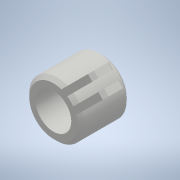
# Autodesk Inventor part: Втулка
Saved by Autodesk Inventor 2020 (Build 240168000, 168)
## iProperties
Created: 2021-05-02
Part Number: Втулка
Material: Типовые
Document SubType Name: Modeling
Designer: I_Love_U_Bogdan
Density: 1 g/cm^3
Appearance: По умолчанию
Author: I_Love_U_Bogdan
Autodesk Inventor part; units mm, degrees
ref_plane "YZ Plane" through (0, 0, 0) normal (1, 0, 0) x (0, 1, 0)
ref_plane "XZ Plane" through (0, 0, 0) normal (0, 1, 0) x (-1, 0, 0)
ref_plane "XY Plane" through (0, 0, 0) normal (0, 0, 1) x (1, 0, 0)
sketch "Эскиз1" plane through (0, 0, 0) normal (0, 0, 1) x (1, 0, 0)
  circle A0 centre (0, 0) radius 8.1 projected
  circle A1 centre (0, 0) radius 8
  circle A2 centre (0, 0) radius 4.6
  dimension "d0" = 0.1
  dimension "d1" = 9.2
  constraints: 2 centre point, 1 coincident
  measures "d0" radial gap between concentric circles of A0 A1
  measures "d1" diameter of A2
extrude "Выдавливание1" add sketch "Эскиз1" along normal blind 14 contours A1
chamfer "Фаска1" distance 1 angle 45 4 edges at (-8, 0, 14) (-8, 0, 0) (-4.6, 0, 14) (-4.6, 0, 0)
sketch "Эскиз2" plane through (0, 0, 14) normal (0, 0, 1) x (1, 0, 0)
  circle A0 centre (15.2735, -186.1533) radius 2.5 projected
  circle A1 centre (19.2813, -181.6882) radius 2.5 projected
  circle A2 centre (6.7164, -177.6929) radius 2.5 projected
  circle A3 centre (6.7164, -107.6929) radius 2.5 projected
  circle A4 centre (11.2658, -120.6185) radius 2.5 projected
  circle A5 centre (6.7164, -37.6929) radius 2.5 projected
  circle A6 centre (15.2735, -46.1533) radius 2.5 projected
  circle A7 centre (23.2891, -37.223) radius 2.5 projected
  circle A8 centre (26, -154.7115) radius 6 projected
  circle A9 centre (26, -84.7115) radius 6 projected
  circle A10 centre (-32.5, -91.359) radius 1.5 projected
  circle A11 centre (-32.5, -21.359) radius 1.5 projected
  line L0 (15.5395, 14.1253) -> (7.4584, 6.0442) projected
  arc A12 (6.0442, 7.4584) -> (7.4584, 6.0442) centre (0, 0) ccw projected
  line L1 (6.0442, 7.4584) -> (14.1253, 15.5395) projected
  arc A13 (14.1253, 15.5395) -> (-20.9712, 1.0986) centre (0, 0) ccw projected
  arc A14 (-25.0526, -8.0684) -> (-20.9712, 1.0986) centre (-34.9521, 1.8311) ccw projected
  line L2 (-25.0526, -8.0684) -> (-27.881, -10.8968) projected
  line L3 (-27.881, -5.24) -> (-27.881, -10.8968) projected
  line L4 (-36.4645, -13.8234) -> (-27.881, -5.24) projected
  line L5 (-39, -19.9448) -> (-36.4645, -13.8234) projected
  line L6 (-39, -107.9932) -> (-39, -19.9448) projected
  line L7 (-38.7059, -110.2271) -> (-39, -107.9932) projected
  line L8 (-11.2941, -212.5294) -> (-38.7059, -110.2271) projected
  line L9 (-10, -222.359) -> (-11.2941, -212.5294) projected
  line L10 (-10, -239.5306) -> (-10, -222.359) projected
  line L11 (-5.9, -243.6306) -> (-10, -239.5306) projected
  line L12 (-5.9, -232.3168) -> (-5.9, -243.6306) projected
  line L13 (-5.9, -232.3168) -> (-1.4533, -236.7636) projected
  arc A15 (-0.3274, -237.8894) -> (-1.4533, -236.7636) centre (0.6355, -235.8007) ccw projected
  line L14 (-0.3274, -237.8894) -> (0.1419, -238.3587) projected
  line L15 (0.1419, -238.3587) -> (21.8181, -232.5506) projected
  arc A16 (21.8181, -232.5506) -> (28.9814, -229.4318) centre (15, -207.1051) ccw projected
  arc A17 (32.6098, -226.6973) -> (28.9814, -229.4318) centre (30.5792, -227.7773) ccw projected
  arc A18 (32.6098, -226.6973) -> (41.3431, -207.1051) centre (15, -207.1051) ccw projected
  line L16 (41.3431, -207.1051) -> (41.3431, -44.3275) projected
  line L17 (40.8708, -43.2834) -> (41.3431, -44.3275) projected
  line L18 (40.8708, -43.2834) -> (30.4465, -37.265) projected
  spline S0 degree 3 poles (30.4465, -37.265) (28.5259, -36.1561) (26.8693, -34.6988) (23.9575, -31.0426) (22.8201, -28.8572) (21.6341, -25.5426) (21.3338, -24.5174) (21.0841, -23.4772) knots -1.71756 -1.71756 -1.71756 -1.71756 -1.05224 -1.05224 -0.317791 -0.317791 0 0 0 0 projected
  arc A19 (20.3792, -6.3803) -> (21.0841, -23.4772) centre (26, -14.7115) ccw projected
  spline S1 degree 3 poles (20.3792, -6.3803) (20.4968, -5.2098) (20.6383, -4.0488) (20.7981, -2.9054) knots -3.756173 -3.756173 -3.756173 -3.756173 -3.409835 -3.409835 -3.409835 -3.409835 projected
  arc A20 (20.7981, -2.9054) -> (15.5395, 14.1253) centre (0, 0) ccw projected
  circle A21 centre (19.2813, -41.6882) radius 2.5 projected
  circle A22 centre (11.2658, -50.6185) radius 2.5 projected
  circle A23 centre (19.2813, -111.6882) radius 2.5 projected
  circle A24 centre (15.2735, -116.1533) radius 2.5 projected
  circle A25 centre (23.2891, -107.223) radius 2.5 projected
  circle A26 centre (23.2891, -177.223) radius 2.5 projected
  circle A27 centre (11.2658, -190.6185) radius 2.5 projected
  circle A28 centre (11.5956, -216.8171) radius 12.85 projected
  circle A29 centre (-7.3879, -205.857) radius 2.3 projected
  circle A30 centre (22.5558, -197.8336) radius 2.3 projected
  circle A31 centre (0, 0) radius 8 projected
  line L19 (2.3508, 6.5935) -> (12.5756, 16.8183)
  line L20 (6.0442, 7.4584) -> (4.1919, 5.6061)
  line L21 (11.9803, 13.3945) -> (10.5661, 14.8088)
  line L22 (10.5661, 11.9803) -> (11.9803, 10.5661)
  circle A32 centre (0, 0) radius 7 projected
  line L23 (0, 0) -> (10.0847, 10.0847)
  line L24 (6.5935, 2.3508) -> (16.8183, 12.5756)
  line L25 (7.4584, 6.0442) -> (5.6061, 4.1919)
  line L26 (13.3945, 11.9803) -> (14.8088, 10.5661)
  line L27 (4.0279, 5.725) -> (11.8389, 13.536)
  line L28 (5.725, 4.0279) -> (13.536, 11.8389)
  point P0 (6.5935, 2.3508)
  dimension "d7" = 2
  dimension "d8" = 2
  dimension "d14" = 0.2
  dimension "d15" = 0.2
  constraints: 20 end point, 5 point on circle, 5 point on line, 5 symmetric about line, 3 perpendicular, 2 parallel, 1 collinear, 3 other
  measures "d7" distance between parallel lines of L21 L22
  measures "d8" distance between parallel lines of L19 L1
  measures "d14" distance between parallel lines of L1 L27
  measures "d15" distance between parallel lines of L0 L28
extrude "Выдавливание2" add sketch "Эскиз2" against normal blind 6 contours L26 L24 A12 L28 | A12 L24 A31 L28 | A31 L24 A32 L28 | L19 L21 L27 A12 | A12 L27 A31 L19 | A31 L27 A32 L19
chamfer "Фаска2" distance 1 angle 45 4 edges at (11.2025, 14.1724, 14) (11.2025, 14.1724, 8) (14.1724, 11.2025, 14) (14.1724, 11.2025, 8)
sketch "Эскиз3" plane through (3.1227, 7.3654, 8) normal (-0.7071, 0.7071, 0) x (-0.7071, -0.7071, 0)
  circle A0 centre (-7.0266, 3.2) radius 1.5 projected
  circle A1 centre (-7.0266, 3.2) radius 1.35
  point P0 (7.4162, -8)
  dimension "d18" = 2.7
  constraints: 1 centre point, 1 coincident
  measures "d18" diameter of A1
extrude "Выдавливание3" cut sketch "Эскиз3" against normal blind 6 contours A1
